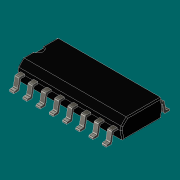
# Autodesk Inventor part: SOIC-16-N
Saved by Autodesk Inventor 2016 (Build 200138000, 138)
## iProperties
Created: 2015-10-12
Part Number: SOIC-16-N
Material: ABS Plastic
Document SubType Name: Modeling
Designer: Sawaiz
Density: 1.06 g/cm^3
Appearance: Smooth - Black
Author: Sawaiz
Autodesk Inventor part; units mm, degrees
ref_plane "YZ Plane" through (0, 0, 0) normal (1, 0, 0) x (0, 1, 0)
ref_plane "XZ Plane" through (0, 0, 0) normal (0, 1, 0) x (-1, 0, 0)
ref_plane "XY Plane" through (0, 0, 0) normal (0, 0, 1) x (1, 0, 0)
sketch "Sketch1" plane through (0, 0, 0) normal (0, 0, 1) x (1, 0, 0)
  line L0 (2, -5) -> (-2, -5)
  line L1 (-2, -5) -> (-2, 5)
  line L2 (-2, 5) -> (2, 5)
  line L3 (2, 5) -> (2, -5)
  line L4 (2, -5) -> (-2, 5) construction
  line L5 (-2, -5) -> (2, 5) construction
  point P0 (0, 0)
  dimension "d0" = 4
  dimension "d1" = 10
  constraints: 12 end point, 2 midpoint, 2 parallel, 1 horizontal, 1 perpendicular
  measures "d0" distance of L1.end L2.end
  measures "d1" distance of L0.end L1.end
extrude "Extrusion1" add sketch "Sketch1" along normal blind 1.72
chamfer "Chamfer1" distance 0.5733 angle 45 1 edges at (2, 0, 1.72)
sketch "Sketch4" plane through (-2, -5, 0) normal (0, -1, 0) x (1, 0, 0)
  line L0 (0, 0) -> (0, 1.72) projected
  line L1 (0, 0.86) -> (4, 0.86)
  line L2 (4, 0) -> (4, 1.1467) projected
  line L3 (0, 0.86) -> (0.1516, 1.72)
  line L4 (0.1516, 1.72) -> (0, 0.86)
  line L5 (0.1516, 0) -> (0, 0.86)
  line L6 (4, 0.86) -> (3.8484, 0)
  line L7 (3.8484, 0) -> (4, 0.86)
  line L8 (3.8484, 1.72) -> (4, 0.86)
  line L9 (4, 0) -> (0, 0) projected
  line L10 (3.8484, 1.72) -> (4, 1.72)
  line L11 (4, 1.72) -> (4, 1.1467)
  line L12 (0, 1.72) -> (3.4267, 1.72) projected
  point P0 (2, 0)
  dimension "d18" = 10
  dimension "d19" = 10
  constraints: 18 end point, 4 equal length, 4 point on line, 2 horizontal, 1 collinear, 1 midpoint, 1 perpendicular
  measures "d18" angle of L0 L3
  measures "d19" angle of L0 L5
extrude "Extrusion2" cut sketch "Sketch4" against normal through all contours L0 L12 L3 | L8 L10 L11 L2 | L0 L5 L9 | L2 L9 L6
ref_plane "Work Plane1" through (-2, -4.6825, 0) normal (0, -1, 0) x (1, 0, 0)
sketch "Sketch2" plane through (-2, -4.6825, 0) normal (0, -1, 0) x (1, 0, 0)
  line L0 (3.4267, 1.72) -> (3.9386, 1.208) projected
  line L1 (0.1516, 1.72) -> (3.4267, 1.72) projected
  line L2 (3.8484, 0) -> (0.1516, 0) projected
  line L3 (3.9824, 0.96) -> (4.525, 0.96)
  line L4 (4.525, 0.96) -> (4.6917, 0.05)
  line L5 (4.6917, 0.05) -> (5.05, 0.05)
  line L6 (5.05, 0.05) -> (5.05, -0.15)
  line L7 (5.05, -0.15) -> (4.525, -0.15)
  line L8 (4.525, -0.15) -> (4.3583, 0.76)
  line L9 (4.3583, 0.76) -> (3.9824, 0.76)
  line L10 (4.525, -0.15) -> (4.525, 0.96)
  line L11 (4, 0.86) -> (3.9386, 1.208) projected
  line L12 (0.1516, 1.72) -> (0, 0.86) projected
  line L13 (0, 0.86) -> (0.1516, 0) projected
  line L14 (3.8484, 0) -> (4, 0.86) projected
  line L15 (4, 0.86) -> (3.9386, 1.208) projected
  line L16 (3.8484, 0) -> (4, 0.86) projected
  dimension "d8" = 0.2
  dimension "d13" = 0.2
  dimension "d15" = 0.2
  dimension "d16" = 0.15
  dimension "d23" = 0.525
  dimension "d24" = 0.525
  dimension "d25" = 0.1
  constraints: 16 end point, 2 parallel, 2 perpendicular, 2 point on line, 1 horizontal, 1 vertical
  measures "d8" distance between parallel lines of L9 L3
  measures "d13" distance between parallel lines of L8 L4
  measures "d15" distance between parallel lines of L5 L7
  measures "d16" distance between parallel lines of L2 L7
  measures "d23" horizontal distance of L11.start L3.end
  measures "d24" distance from line of L3.end L6
  measures "d25" distance from line of L3 L15.start
extrude "Extrusion3" add sketch "Sketch2" against normal blind 0.4
fillet "Fillet1" radius 0.1 5 edges at (2.525, -4.4825, 0.96) (2.6917, -4.4825, 0.05) (3.05, -4.4825, 0.05) (2.525, -4.4825, -0.15) (2.3583, -4.4825, 0.76)
pattern_linear "Rectangular Pattern1" count 8 spacing 1.27 along (0, 1, 0) of "Extrusion3", "Fillet1"
mirror "Mirror1" about plane through (0, 0, 0) normal (1, 0, 0) of "Extrusion3", "Fillet1", "Rectangular Pattern1"
sketch "Sketch5" plane through (-1.8484, -5, 0) normal (0, -1, 0) x (1, 0, 0)
  line L0 (3.787, 1.208) -> (3.275, 1.72) projected
  line L1 (3.6967, 1.72) -> (3.787, 1.208) projected
  line L2 (3.275, 1.72) -> (3.6967, 1.72) projected
  point P0 (1.8484, 0)
extrude "Extrusion4" cut sketch "Sketch5" against normal through all
sketch "Sketch6" plane through (0, 0, 1.72) normal (0, 0, 1) x (1, 0, 0)
  line L0 (1.4267, 5) -> (1.4267, -5) projected
  line L1 (1.4267, 5) -> (-1.8484, 5) projected
  line L2 (-1.8484, 5) -> (-1.8484, -5) projected
  line L3 (-1.8484, -5) -> (1.4267, -5) projected
  line L4 (-1.8484, -5) -> (1.4267, -5) projected
  circle A0 centre (0, -5) radius 0.5
  line L5 (-2, -4.6825) -> (-2, -5) projected
  point P0 (0, 0)
  dimension "d34" = 1
  dimension "d38" = 2
  constraints: 1 centre point, 1 point on line
  measures "d34" diameter of A0
  measures "d38" distance from line of L5 A0.centre
extrude "Extrusion5" cut sketch "Sketch6" against normal blind 0.215 contours A0 L3 | L3 A0
fillet "Fillet2" radius 0.1075 15 edges at (-0.2108, 5, 1.72) (1.6826, 5, 1.464) (1.9693, 5, 1.034) (1.9242, 5, 0.43) (0, 5, 0) (-1.9242, 5, 0.43) (-1.9242, 5, 1.29) (-1.1742, -5, 1.72) (0.9633, -5, 1.72) (1.6826, -5, 1.464) (1.9693, -5, 1.034) (1.9242, -5, 0.43) (0, -5, 0) (-1.9242, -5, 0.43) (-1.9242, -5, 1.29)
equation "\"d0\" = bodyWidth"
equation "\"d1\" = length"
equation "\"d2\" = height"
equation "\"d4\" = 0.333333 * height"
equation "\"d21\" = height"
equation "\"d8\" = leadThickness"
equation "\"d13\" = leadThickness"
equation "\"d15\" = leadThickness"
equation "\"d16\" = clearence"
equation "\"d23\" = 0.5 * leadLength"
equation "\"d24\" = 0.5 * leadLength"
equation "\"d25\" = 0.5 * leadThickness"
equation "\"d26\" = leadWidth"
equation "\"d28\" = 0.5 * leadThickness"
equation "\"d31\" = pitch"
equation "\"d32\" = leadWidth"
equation "\"d34\" = 0.25 * bodyWidth"
equation "\"d38\" = 0.5 * bodyWidth"
equation "\"d35\" = 0.125 * height"
equation "\"d37\" = 0.0625 * height"
equation "\"clearence\" = 0.15"
equation "\"height\" = 1.72"
equation "\"leadThickness\" = 0.2"
equation "\"length\" = 10"
equation "\"leadWidth\" = 0.4"
equation "\"leadLength\" = 1.05"
equation "\"pitch\" = 1.27"
equation "\"bodyWidth\" = 4"
equation "\"leadToLeadWidth\" = 6"
equation "\"d7\" = -0.25 * pitch"
body "Solid1"
